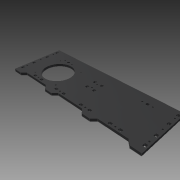
# Autodesk Inventor part: back
Saved by Autodesk Inventor 2014 (Build 180170000, 170)
## iProperties
Created: 2013-12-05
Part Number: back
Material: Generic
Document SubType Name: Modeling
Designer: buben
Density: 1 g/cm^3
Appearance: Anodized - Dark Gray
Author: buben
Subject: Laser Cutted
Autodesk Inventor part; units mm, degrees
ref_plane "YZ Plane" through (0, 0, 0) normal (1, 0, 0) x (0, 1, 0)
ref_plane "XZ Plane" through (0, 0, 0) normal (0, 1, 0) x (-1, 0, 0)
ref_plane "XY Plane" through (0, 0, 0) normal (0, 0, 1) x (1, 0, 0)
sketch "Sketch1" plane through (0, 0, 0) normal (0, 0, 1) x (1, 0, 0)
  line L0 (0, 0) -> (354, 0)
  line L1 (354, 0) -> (354, 120.5)
  line L2 (354, 120.5) -> (0, 120.5)
  line L3 (0, 120.5) -> (0, 0)
  dimension "d0" = 120.5
  dimension "d1" = 354
  constraints: 8 end point, 2 parallel, 1 horizontal, 1 perpendicular
  measures "d0" distance of L2.end L0.start
  measures "d1" distance of L0.start L0.end
extrude "Extrusion1" add sketch "Sketch1" along normal blind 6.5
sketch "Sketch3" plane through (0, 0, 6.5) normal (0, 0, 1) x (1, 0, 0)
  line L0 (0, 0) -> (354, 0) projected
  line L1 (354, 120.5) -> (0, 120.5) projected
  line L2 (0, 120.5) -> (0, 0) projected
  circle A0 centre (64, 96) radius 4
  circle A1 centre (290, 96) radius 4
  line L3 (64, 96) -> (290, 96) construction
  point P0 (177, 96)
  point P1 (177, 120.5)
  dimension "d9" = 8
  dimension "d10" = 96
  dimension "d11" = 226
  constraints: 2 centre point, 2 end point, 2 midpoint, 1 equal radius, 1 horizontal alignment, 1 perpendicular, 1 vertical alignment
  measures "d9" diameter of A0
  measures "d10" distance from line of L0 L3.start
  measures "d11" distance of L3.start L3.end
extrude "Extrusion3" cut sketch "Sketch3" against normal through all
sketch "Sketch4" plane through (0, 0, 6.5) normal (0, 0, 1) x (1, 0, 0)
  line L0 (0, 0) -> (354, 0) projected
  line L1 (354, 120.5) -> (0, 120.5) projected
  line L2 (0, 120.5) -> (0, 0) projected
  circle A0 centre (6.25, 18.5) radius 2.25
  circle A1 centre (6.25, 57.5) radius 2.25
  circle A2 centre (6.25, 96.5) radius 2.25
  line L3 (177, 120.5) -> (177, 0) construction
  line L4 (3, 112) -> (9.5, 112)
  line L5 (9.5, 112) -> (9.5, 104)
  line L6 (9.5, 104) -> (3, 104)
  line L7 (3, 104) -> (3, 112)
  line L8 (3, 81) -> (9.5, 81)
  line L9 (9.5, 81) -> (9.5, 73)
  line L10 (9.5, 73) -> (3, 73)
  line L11 (3, 73) -> (3, 81)
  line L12 (3, 42) -> (9.5, 42)
  line L13 (9.5, 42) -> (9.5, 34)
  line L14 (9.5, 34) -> (3, 34)
  line L15 (3, 34) -> (3, 42)
  line L16 (3, 11) -> (9.5, 11)
  line L17 (9.5, 11) -> (9.5, 3)
  line L18 (9.5, 3) -> (3, 3)
  line L19 (3, 3) -> (3, 11)
  line L20 (6.25, 18.5) -> (6.25, 57.5) construction
  line L21 (6.25, 57.5) -> (6.25, 96.5) construction
  circle A3 centre (347.75, 18.5) radius 2.25
  circle A4 centre (347.75, 57.5) radius 2.25
  circle A5 centre (347.75, 96.5) radius 2.25
  line L22 (351, 112) -> (344.5, 112)
  line L23 (344.5, 112) -> (344.5, 104)
  line L24 (344.5, 104) -> (351, 104)
  line L25 (351, 104) -> (351, 112)
  line L26 (351, 81) -> (344.5, 81)
  line L27 (344.5, 81) -> (344.5, 73)
  line L28 (344.5, 73) -> (351, 73)
  line L29 (351, 73) -> (351, 81)
  line L30 (351, 42) -> (344.5, 42)
  line L31 (344.5, 42) -> (344.5, 34)
  line L32 (344.5, 34) -> (351, 34)
  line L33 (351, 34) -> (351, 42)
  line L34 (351, 11) -> (344.5, 11)
  line L35 (344.5, 11) -> (344.5, 3)
  line L36 (344.5, 3) -> (351, 3)
  line L37 (351, 3) -> (351, 11)
  line L38 (347.75, 18.5) -> (347.75, 57.5) construction
  line L39 (347.75, 57.5) -> (347.75, 96.5) construction
  point P0 (6.25, 104)
  point P1 (3, 38)
  point P2 (6.25, 38)
  point P3 (3, 77)
  point P4 (6.25, 77)
  point P5 (347.75, 104)
  point P6 (351, 38)
  point P7 (347.75, 38)
  point P8 (351, 77)
  point P9 (347.75, 77)
  dimension "d14" = 18.5
  dimension "d15" = 39
  dimension "d16" = 39
  dimension "d17" = 4.5
  dimension "d18" = 6.5
  dimension "d19" = 8
  dimension "d20" = 8
  dimension "d21" = 8
  dimension "d22" = 8
  dimension "d23" = 3
  dimension "d27" = 23
  dimension "d28" = 3
  constraints: 74 end point, 24 symmetric about line, 9 parallel, 7 collinear, 7 midpoint, 6 centre point, 4 horizontal, 4 perpendicular, 3 vertical alignment, 2 equal radius, 2 horizontal alignment, 3 other
  measures "d14" distance from line of L0 L20.start
  measures "d15" distance of L20.start L20.end
  measures "d16" distance of L20.end L21.end
  measures "d17" diameter of A0
  measures "d18" distance of L4.start L4.end
  measures "d19" distance of L6.end L4.start
  measures "d20" distance of L10.end L8.start
  measures "d21" distance of L14.end L12.start
  measures "d22" distance of L18.end L16.start
  measures "d23" distance between parallel lines of L0 L18
  measures "d27" distance between parallel lines of L8 L6
  measures "d28" distance between parallel lines of L2 L7
extrude "Extrusion4" cut sketch "Sketch4" against normal through all
sketch "Sketch5" plane through (0, 0, 6.5) normal (0, 0, 1) x (1, 0, 0)
  line L0 (0, 0) -> (354, 0) projected
  line L1 (51.7, 9.5) -> (59.7, 9.5)
  line L2 (59.7, 9.5) -> (59.7, 3)
  line L3 (59.7, 3) -> (51.7, 3)
  line L4 (51.7, 3) -> (51.7, 9.5)
  line L5 (74.7, 9.5) -> (82.7, 9.5)
  line L6 (82.7, 9.5) -> (82.7, 3)
  line L7 (82.7, 3) -> (74.7, 3)
  line L8 (74.7, 3) -> (74.7, 9.5)
  line L9 (59.7, 9.5) -> (74.7, 3) construction
  line L10 (74.7, 9.5) -> (59.7, 3) construction
  circle A0 centre (67.2, 6.25) radius 2.25
  line L11 (124.9, 9.5) -> (132.9, 9.5)
  line L12 (132.9, 9.5) -> (132.9, 3)
  line L13 (132.9, 3) -> (124.9, 3)
  line L14 (124.9, 3) -> (124.9, 9.5)
  line L15 (147.9, 9.5) -> (155.9, 9.5)
  line L16 (155.9, 9.5) -> (155.9, 3)
  line L17 (155.9, 3) -> (147.9, 3)
  line L18 (147.9, 3) -> (147.9, 9.5)
  line L19 (132.9, 9.5) -> (147.9, 3) construction
  line L20 (147.9, 9.5) -> (132.9, 3) construction
  circle A1 centre (140.4, 6.25) radius 2.25
  line L21 (198.1, 9.5) -> (206.1, 9.5)
  line L22 (206.1, 9.5) -> (206.1, 3)
  line L23 (206.1, 3) -> (198.1, 3)
  line L24 (198.1, 3) -> (198.1, 9.5)
  line L25 (221.1, 9.5) -> (229.1, 9.5)
  line L26 (229.1, 9.5) -> (229.1, 3)
  line L27 (229.1, 3) -> (221.1, 3)
  line L28 (221.1, 3) -> (221.1, 9.5)
  line L29 (206.1, 9.5) -> (221.1, 3) construction
  line L30 (221.1, 9.5) -> (206.1, 3) construction
  circle A2 centre (213.6, 6.25) radius 2.25
  line L31 (271.3, 9.5) -> (279.3, 9.5)
  line L32 (279.3, 9.5) -> (279.3, 3)
  line L33 (279.3, 3) -> (271.3, 3)
  line L34 (271.3, 3) -> (271.3, 9.5)
  line L35 (294.3, 9.5) -> (302.3, 9.5)
  line L36 (302.3, 9.5) -> (302.3, 3)
  line L37 (302.3, 3) -> (294.3, 3)
  line L38 (294.3, 3) -> (294.3, 9.5)
  line L39 (279.3, 9.5) -> (294.3, 3) construction
  line L40 (294.3, 9.5) -> (279.3, 3) construction
  circle A3 centre (286.8, 6.25) radius 2.25
  line L41 (51.7, 6.25) -> (9.5, 6.25) construction
  line L42 (82.7, 6.25) -> (124.9, 6.25) construction
  line L43 (155.9, 6.25) -> (198.1, 6.25) construction
  line L44 (229.1, 6.25) -> (271.3, 6.25) construction
  line L45 (302.3, 6.25) -> (344.5, 6.25) construction
  point P0 (9.5, 3)
  point P1 (344.5, 3)
  point P2 (286.8, 6.25)
  dimension "d31" = 8
  dimension "d32" = 6.5
  dimension "d33" = 8
  dimension "d34" = 15
  dimension "d35" = 4.5
  dimension "d36" = 8
  dimension "d37" = 6.5
  dimension "d38" = 8
  dimension "d39" = 15
  dimension "d40" = 4.5
  dimension "d41" = 8
  dimension "d42" = 6.5
  dimension "d43" = 8
  dimension "d44" = 15
  dimension "d45" = 4.5
  dimension "d46" = 8
  dimension "d47" = 6.5
  dimension "d48" = 8
  dimension "d49" = 15
  dimension "d50" = 4.5
  dimension "d51" = 3
  constraints: 90 end point, 17 parallel, 13 collinear, 13 midpoint, 8 horizontal, 8 perpendicular, 4 centre point, 3 horizontal alignment, 2 vertical alignment
  measures "d31" distance of L1.start L1.end
  measures "d32" distance of L3.end L1.start
  measures "d33" distance of L5.start L5.end
  measures "d34" distance between parallel lines of L8 L2
  measures "d35" diameter of A0
  measures "d36" distance of L14.end L11.end
  measures "d37" distance of L14.start L14.end
  measures "d38" distance of L20.start L15.end
  measures "d39" distance between parallel lines of L18 L12
  measures "d40" diameter of A1
  measures "d41" distance of L24.end L21.end
  measures "d42" distance of L24.start L24.end
  measures "d43" distance of L30.start L25.end
  measures "d44" distance between parallel lines of L28 L22
  measures "d45" diameter of A2
  measures "d46" distance of L34.end L31.end
  measures "d47" distance of L34.start L34.end
  measures "d48" distance of L40.start L35.end
  measures "d49" distance between parallel lines of L38 L32
  measures "d50" diameter of A3
  measures "d51" distance between parallel lines of L0 L3
extrude "Extrusion5" cut sketch "Sketch5" against normal through all
sketch "Sketch6" plane through (0, 0, 6.5) normal (0, 0, 1) x (1, 0, 0)
  line L0 (0, 0) -> (354, 0) projected
  line L1 (0, 120.5) -> (0, 0) projected
  line L2 (0, 0) -> (0, -10)
  line L3 (0, -10) -> (23, -10)
  line L4 (23, -10) -> (33, 0)
  line L5 (102.3333, 0) -> (112.3333, -10)
  line L6 (112.3333, -10) -> (132.3333, -10)
  line L7 (132.3333, -10) -> (142.3333, 0)
  line L8 (211.6667, 0) -> (221.6667, -10)
  line L9 (221.6667, -10) -> (241.6667, -10)
  line L10 (241.6667, -10) -> (251.6667, 0)
  line L11 (354, 0) -> (354, -10)
  line L12 (354, -10) -> (331, -10)
  line L13 (331, -10) -> (321, 0)
  line L14 (23, -10) -> (112.3333, -10) construction
  line L15 (132.3333, -10) -> (221.6667, -10) construction
  line L16 (241.6667, -10) -> (331, -10) construction
  dimension "d54" = 20
  dimension "d55" = 23
  dimension "d56" = 45
  dimension "d57" = 10
  constraints: 30 end point, 13 collinear, 8 perpendicular, 6 point on line
  measures "d54" distance of L5.end L6.end
  measures "d55" distance of L2.end L3.end
  measures "d56" angle of L4 L3
  measures "d57" distance of L0.start L2.end
extrude "Extrusion6" add sketch "Sketch6" against normal blind 6.5
sketch "Sketch7" plane through (0, 0, 6.5) normal (0, 0, 1) x (1, 0, 0)
  line L0 (354, 120.5) -> (0, 120.5) projected
  line L1 (173.5, 81.6) -> (180.5, 81.6) construction
  line L2 (180.5, 81.6) -> (180.5, 55.6) construction
  line L3 (180.5, 55.6) -> (173.5, 55.6) construction
  line L4 (173.5, 55.6) -> (173.5, 81.6) construction
  line L5 (183.75, 84.1) -> (190.25, 84.1)
  line L6 (190.25, 84.1) -> (190.25, 76.1)
  line L7 (190.25, 76.1) -> (183.75, 76.1)
  line L8 (183.75, 76.1) -> (183.75, 84.1)
  line L9 (183.75, 61.1) -> (190.25, 61.1)
  line L10 (190.25, 61.1) -> (190.25, 53.1)
  line L11 (190.25, 53.1) -> (183.75, 53.1)
  line L12 (183.75, 53.1) -> (183.75, 61.1)
  line L13 (163.75, 84.1) -> (170.25, 84.1)
  line L14 (170.25, 84.1) -> (170.25, 76.1)
  line L15 (170.25, 76.1) -> (163.75, 76.1)
  line L16 (163.75, 76.1) -> (163.75, 84.1)
  line L17 (163.75, 61.1) -> (170.25, 61.1)
  line L18 (170.25, 61.1) -> (170.25, 53.1)
  line L19 (170.25, 53.1) -> (163.75, 53.1)
  line L20 (163.75, 53.1) -> (163.75, 61.1)
  line L21 (170.25, 76.1) -> (183.75, 61.1) construction
  line L22 (183.75, 76.1) -> (170.25, 61.1) construction
  circle A0 centre (177, 76.1) radius 2.25
  circle A1 centre (177, 61.1) radius 2.25
  line L23 (177, 76.1) -> (177, 61.1) construction
  point P0 (147.9, 9.5)
  point P1 (0, 0)
  point P2 (177, 81.6)
  point P3 (177, 120.5)
  point P4 (177, 68.6)
  point P5 (173.5, 68.6)
  point P6 (177, 68.6)
  dimension "d60" = 7
  dimension "d61" = 26
  dimension "d62" = 72.1
  dimension "d63" = 8
  dimension "d64" = 6.5
  dimension "d65" = 6.5
  dimension "d66" = 8
  dimension "d67" = 13.5
  dimension "d68" = 15
  dimension "d69" = 4.5
  dimension "d70" = 15
  constraints: 46 end point, 11 parallel, 8 collinear, 6 midpoint, 5 horizontal, 5 perpendicular, 3 vertical alignment, 2 centre point, 1 equal radius, 1 horizontal alignment
  measures "d60" distance of L1.start L1.end
  measures "d61" distance of L3.end L1.start
  measures "d62" vertical distance of point (177, 81.6) point (147.9, 9.5)
  measures "d63" distance of L15.end L13.start
  measures "d64" distance of L13.start L13.end
  measures "d65" distance of L5.start L5.end
  measures "d66" distance of L19.end L17.start
  measures "d67" distance between parallel lines of L8 L14
  measures "d68" distance between parallel lines of L9 L7
  measures "d69" diameter of A0
  measures "d70" distance of L23.start L23.end
extrude "Extrusion7" cut sketch "Sketch7" against normal through all
sketch "Sketch8" plane through (0, 0, 6.5) normal (0, 0, 1) x (1, 0, 0)
  line L0 (163.75, 84.1) -> (170.25, 84.1) projected
  circle A0 centre (64, 96) radius 4 projected
  circle A1 centre (290, 96) radius 4 projected
  line L1 (354, 120.5) -> (0, 120.5) projected
  circle A2 centre (52, 96) radius 2.25
  circle A3 centre (76, 96) radius 2.25
  circle A4 centre (278, 96) radius 2.25
  circle A5 centre (302, 96) radius 2.25
  line L2 (52, 96) -> (76, 96) construction
  line L3 (278, 96) -> (302, 96) construction
  point P0 (0, 0)
  dimension "d73" = 24
  dimension "d74" = 4.5
  constraints: 4 centre point, 4 end point, 3 equal radius, 2 coincident, 2 collinear, 2 midpoint, 2 parallel
  measures "d73" distance of L2.start L2.end
  measures "d74" diameter of A2
extrude "Extrusion8" cut sketch "Sketch8" against normal through all contours A2 | A3 | A4 | A5
sketch "Sketch9" plane through (0, 0, 6.5) normal (0, 0, 1) x (1, 0, 0)
  line L0 (74.7, 9.5) -> (82.7, 9.5) projected
  line L1 (9.5, 42) -> (9.5, 34) projected
  line L2 (44.5, 87) -> (117, 87) construction
  line L3 (117, 87) -> (117, 14.5) construction
  line L4 (117, 14.5) -> (44.5, 14.5) construction
  line L5 (44.5, 14.5) -> (44.5, 87) construction
  circle A0 centre (44.5, 87) radius 2
  circle A1 centre (117, 87) radius 2
  circle A2 centre (117, 14.5) radius 2
  circle A3 centre (44.5, 14.5) radius 2
  line L6 (40.75, 90.75) -> (120.75, 90.75) construction
  line L7 (120.75, 90.75) -> (120.75, 10.75) construction
  line L8 (120.75, 10.75) -> (40.75, 10.75) construction
  line L9 (40.75, 10.75) -> (40.75, 90.75) construction
  point P0 (0, 0)
  point P1 (80.75, 10.75)
  point P2 (80.75, 14.5)
  point P3 (40.75, 50.75)
  point P4 (44.5, 50.75)
  dimension "d77" = 4
  dimension "d78" = 72.5
  dimension "d79" = 5
  dimension "d80" = 80
  dimension "d81" = 35
  constraints: 16 end point, 4 centre point, 4 coincident, 4 midpoint, 4 parallel, 4 perpendicular, 3 equal radius, 2 horizontal, 1 horizontal alignment, 1 vertical alignment
  measures "d77" diameter of A3
  measures "d78" distance of L4.end L2.start
  measures "d79" distance between parallel lines of L0 L4
  measures "d80" distance of L7.end L8.end
  measures "d81" distance between parallel lines of L1 L5
extrude "Extrusion9" cut sketch "Sketch9" against normal through all
sketch "Sketch10" plane through (0, 0, 6.5) normal (0, 0, 1) x (1, 0, 0)
  circle A0 centre (117, 14.5) radius 2 projected
  circle A1 centre (44.5, 87) radius 2 projected
  line L0 (44.5, 87) -> (117, 87) construction
  line L1 (117, 87) -> (117, 14.5) construction
  line L2 (117, 14.5) -> (44.5, 14.5) construction
  line L3 (44.5, 14.5) -> (44.5, 87) construction
  circle A2 centre (80.75, 50.75) radius 37.5
  line L4 (40.75, 98.6417) -> (120.75, 98.6417)
  line L5 (120.75, 98.6417) -> (120.75, 18.6417)
  line L6 (120.75, 18.6417) -> (40.75, 18.6417)
  line L7 (40.75, 18.6417) -> (40.75, 98.6417)
  point P0 (0, 0)
  point P1 (80.75, 87)
  point P2 (44.5, 50.75)
  point P3 (80.75, 98.6417)
  dimension "d84" = 75
  dimension "d87" = 80
  constraints: 16 end point, 4 parallel, 3 midpoint, 3 perpendicular, 2 coincident, 2 horizontal, 2 vertical alignment, 1 centre point, 1 horizontal alignment
  measures "d84" diameter of A2
  measures "d87" distance of L4.start L4.end
extrude "Extrusion10" cut sketch "Sketch10" against normal through all contours A2 L6 | L6 A2
body "Solid1"
